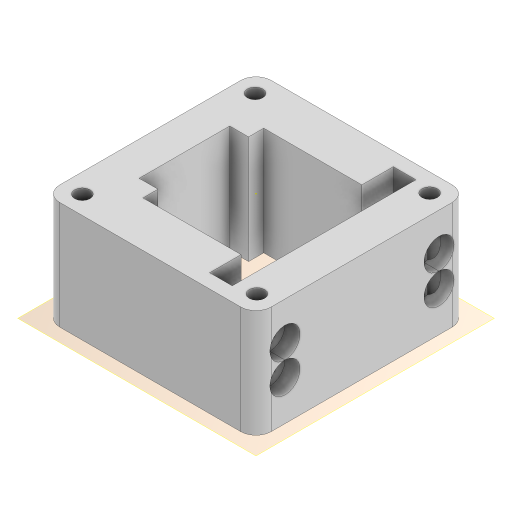
# Autodesk Inventor part: 00_Micro_Stepper_15mm_Gearbox_NEMA17Adapter
Saved by Autodesk Inventor 2024.1 (Build 281209000, 209)
## iProperties
Created: 2024-08-29
Part Number: 00_Micro_Stepper_15mm_Gearbox_NEMA17Adapter
Material: Generisch
Document SubType Name: Modeling
Designer: diederichbenedict
Density: 1 g/cm^3
Appearance: Vorgabe
Author: diederichbenedict
Autodesk Inventor part; units mm, degrees
ref_plane "YZ Plane" through (0, 0, 0) normal (1, 0, 0) x (0, 1, 0)
ref_plane "XZ Plane" through (0, 0, 0) normal (0, 1, 0) x (-1, 0, 0)
ref_plane "Arbeitsebene1" through (0, 0, 0) normal (0, 0, 1) x (1, 0, 0)
sketch "Skizze1" plane through (0, 0, 0) normal (0, 0, 1) x (1, 0, 0)
  line L0 (9.3361, 9.0616) -> (14.1886, 9.0946) projected
  line L1 (14.1529, 14.3445) -> (14.1886, 9.0946) projected
  line L2 (-14.3464, 14.1509) -> (14.1529, 14.3445) projected
  line L3 (-14.1529, -14.3445) -> (-14.3464, 14.1509) projected
  line L4 (14.3464, -14.1509) -> (-14.1529, -14.3445) projected
  line L5 (14.3108, -8.905) -> (14.3464, -14.1509) projected
  line L6 (14.3108, -8.905) -> (9.4584, -8.938) projected
  line L7 (9.4584, -8.938) -> (9.4533, -8.1804) projected
  arc A0 (9.3413, 8.3041) -> (9.4533, -8.1804) centre (0, -0.002) ccw projected
  line L8 (9.3413, 8.3041) -> (9.3361, 9.0616) projected
  circle A1 centre (-11.5623, 11.4353) radius 1.025 projected
  circle A2 centre (-11.4373, -11.5643) radius 1.025 projected
  circle A3 centre (11.5623, -11.4393) radius 1.025 projected
  circle A4 centre (11.4374, 11.5603) radius 1.025 projected
  line L9 (14.1886, 9.0946) -> (14.3108, -8.905)
  line L10 (-12, -14.002) -> (12, -14.002)
  line L11 (14, -12.002) -> (14, 11.998)
  line L12 (12, 13.998) -> (-12, 13.998)
  line L13 (-14, 11.998) -> (-14, -12.002)
  line L14 (-14, -14.002) -> (14, 13.998) construction
  line L15 (14, -14.002) -> (-14, 13.998) construction
  arc A5 (14, 11.998) -> (12, 13.998) centre (12, 11.998) ccw
  arc A6 (12, -14.002) -> (14, -12.002) centre (12, -12.002) ccw
  arc A7 (-14, -12.002) -> (-12, -14.002) centre (-12, -12.002) ccw
  arc A8 (-12, 13.998) -> (-14, 11.998) centre (-12, 11.998) ccw
  circle A9 centre (0, -0.002) radius 5
  point P0 (0, 0)
  dimension "d0" = 28
  dimension "d1" = 28
  dimension "d2" = 2
  dimension "d3" = 10
  constraints: 14 end point, 8 point on circle, 8 point on line, 8 tangent, 5 centre point, 3 equal radius, 2 midpoint, 2 parallel, 2 perpendicular, 1 coincident, 1 horizontal
  measures "d0" distance of L15.end L14.end
  measures "d1" distance of L14.end L15.start
  measures "d2" radius of A5
  measures "d3" diameter of A9
ref_plane "Arbeitsebene2" through (-46.5464, -55.86, 14.3) normal (0, 0, 1) x (1, 0, 0)
extrude "Extrusion1" add sketch "Skizze1" along normal up to surface (14.3 mm away) contours L8 A0 L7 L6 L11 A6 L10 A7 L13 A8 L12 A5 L0 | L0 L11 L6 L7 A0 L8
sketch "Skizze2" plane through (-12, 13.998, 14.3) normal (0, 0, 1) x (1, 0, 0)
  line L0 (21, -26.144) -> (18.4343, -26.144)
  line L1 (16.9611, -1.8095) -> (21, -1.8095)
  line L2 (21, -1.8095) -> (21, -26.144)
  line L3 (21, -5.9767) -> (5, -5.9767)
  line L4 (5, -5.9767) -> (5, -21.9767)
  line L5 (5, -21.9767) -> (21, -21.9767)
  line L6 (21, -21.9767) -> (21, -5.9767)
  line L7 (21, -26.144) -> (18, -26.144)
  line L8 (18, -26.144) -> (18, -1.7609)
  line L9 (18, -1.7609) -> (21, -1.7609)
  line L10 (21, -1.7609) -> (21, -26.144)
  circle A0 centre (12, -14) radius 5 projected
  line L11 (7.5, -7.9767) -> (2.5, -7.9767)
  line L12 (2.5, -7.9767) -> (2.5, -19.9767)
  line L13 (2.5, -19.9767) -> (7.5, -19.9767)
  line L14 (7.5, -19.9767) -> (7.5, -7.9767)
  line L15 (7.5, -7.9767) -> (2.5, -19.9767) construction
  line L16 (2.5, -7.9767) -> (7.5, -19.9767) construction
  point P0 (21, -13.9767)
  point P1 (5, -13.9767)
  point P2 (5, -19.9767)
  point P3 (18, -21.9767)
  point P4 (18, -1.8095)
  point P5 (18, -5.9767)
  point P6 (5, -7.9767)
  dimension "d19" = 16
  dimension "d20" = 16
  dimension "d21" = 3
  dimension "d22" = 9
  dimension "d23" = 9
  dimension "d24" = 5
  dimension "d25" = 12
  constraints: 34 end point, 7 parallel, 5 midpoint, 4 horizontal, 3 perpendicular
  measures "d19" distance of L5.end L4.end
  measures "d20" distance of L4.end L3.end
  measures "d21" distance of L8.end L9.end
  measures "d22" distance from line of L2 A0.centre
  measures "d23" horizontal distance of A0.centre L0.start
  measures "d24" distance of L13.end L12.end
  measures "d25" distance of L12.end L11.end
extrude "Extrusion2" cut sketch "Skizze2" against normal up to surface (14.3 mm away) contours L0 L7 L8 L5 L2 | L5 L8 L3 L2 | L3 L8 L1 L2 | L5 L4 L13 L14 A0 L11 L3 L8 | L13 L12 L11 L4 | L4 L11 L14 A0 L13
sketch "Skizze3" plane through (14, -12.002, 0) normal (1, 0, 0) x (0, 0, -1)
  ellipse E0 centre (-9.3, 22.2405) end of major axis (-8.8, 22.2405) minor radius 0.5 projected
  ellipse E1 centre (-9.3, 1.841) end of major axis (-8.8, 1.841) minor radius 0.5 projected
  ellipse E2 centre (-5.3, 22.2405) end of major axis (-4.8, 22.2405) minor radius 0.5 projected
  ellipse E3 centre (-1.3, 1.841) end of major axis (-0.8, 1.841) minor radius 0.5 projected
  ellipse E4 centre (-5.3, 1.841) end of major axis (-4.8, 1.841) minor radius 0.5 projected
  ellipse E5 centre (-1.3, 22.2405) end of major axis (-0.8, 22.2405) minor radius 0.5 projected
  line L0 (-0.8, 19.7906) -> (-14.3, 19.7906) projected
  line L1 (-14.3, 24.0405) -> (-14.3, 19.7906) projected
  line L2 (1.7, 24.0405) -> (-14.3, 24.0405) projected
  line L3 (1.7, 0.041) -> (1.7, 24.0405) projected
  line L4 (-14.3, 0.041) -> (1.7, 0.041) projected
  line L5 (-14.3, 4.2909) -> (-14.3, 0.041) projected
  line L6 (-14.3, 4.2909) -> (-0.8, 4.2909) projected
  line L7 (-0.8, 4.2909) -> (-0.8, 19.7906) projected
  point P0 (0, 12.002)
hole "Bohrung1" at (14, 10.2385, 5.3) at (14, 10.2385, 9.3) at (14, -10.161, 5.3) at (14, -10.161, 9.3) direction (-1, 0, 0) diameter 1.8 end through all counterbore diameter 4 counterbore depth 2
sketch "Skizze4" plane through (-12, 13.998, 14.3) normal (0, 0, 1) x (1, 0, 0)
  point P0 (12, -13.998)
